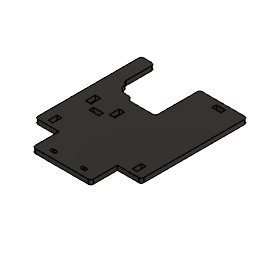
つくプロ (Autodesk Fusion 360 design; units mm, degrees)
Autodesk Fusion 360 part; units mm, degrees
sketch "スケッチ1" plane through (0, 0, 0) normal (0, 0, 1) x (1, 0, 0)
  line L0 (-60, 15) -> (-60, 150)
  line L1 (0, 165) -> (0, 0)
  line L2 (60, 15) -> (60, 150)
  line L3 (-60, 150) -> (-60, 165)
  line L4 (-60, 165) -> (60, 165)
  line L5 (60, 165) -> (60, 150)
  line L6 (-60, 15) -> (60, 15)
  dimension "d20" = 15
  constraint vertical L0
  constraint vertical L1
  constraint coincident L1.end origin
  constraint symmetric L0.end L1 L2.end
  constraint vertical L3
  constraint horizontal L4
  constraint vertical L5
  constraint midpoint L1.start L4
  constraint horizontal L6
  measures "d20" distance of L2.end L4.end
extrude "押し出し1" add sketch "スケッチ1" along normal blind 5
sketch "スケッチ2" plane through (0, 0, 5) normal (0, 0, 1) x (-1, 0, 0)
  line L0 (-60, -15) -> (-60, -165)
  line L1 (60, -165) -> (60, -15)
  line L2 (60, -15) -> (33, -15)
  line L3 (33, -15) -> (33, -45)
  line L4 (33, -45) -> (60, -45)
  line L5 (60, -45) -> (60, -15)
  line L6 (0, -150) -> (0, 0)
  line L7 (-33, -45) -> (-60, -45)
  line L8 (-60, -45) -> (-60, -15)
  line L9 (-60, -15) -> (-33, -15)
  line L10 (-33, -15) -> (-33, -45)
  line L11 (45, -73.5175) -> (45, 1.4825)
  line L12 (60, -15) -> (-60, -15)
  line L13 (-60, -165) -> (60, -165)
  dimension "d38" = 27
  constraint horizontal L2
  constraint vertical L3
  constraint horizontal L4
  constraint vertical L5
  constraint coincident L1 L2.start
  constraint coincident L6.end origin
  constraint symmetric L1.end L6 L0.start
  constraint symmetric L2.end L6 L9.end
  measures "d38" distance of L3 L5
extrude "押し出し2" cut sketch "スケッチ2" against normal blind 35 contours L0 L7 L8 L9 L10 L12 | L2 L3 L4 L11 L12 | L1 L2 L4 L5 L11 L12
fillet "フィレット1" radius 3 6 edges at (60, 45, 2.5) (60, 165, 2.5) (-60, 165, 2.5) (-60, 45, 2.5) (-33, 15, 2.5) (33, 15, 2.5)
sketch "スケッチ16" plane through (0, 0, 5) normal (0, 0, 1) x (-1, 0, 0)
  arc A0 (-30, -15) -> (-33, -18) centre (-30, -18) ccw
  line L0 (-33, -18) -> (-33, -45)
  line L1 (-33, -45) -> (-57, -45)
  arc A1 (-57, -45) -> (-60, -48) centre (-57, -48) ccw
  line L2 (-60, -48) -> (-60, -162)
  arc A2 (-60, -162) -> (-57, -165) centre (-57, -162) ccw
  line L3 (-57, -165) -> (57, -165)
  arc A3 (57, -165) -> (60, -162) centre (57, -162) ccw
  line L4 (60, -162) -> (60, -48)
  arc A4 (60, -48) -> (57, -45) centre (57, -48) ccw
  line L5 (57, -45) -> (33, -45)
  line L6 (33, -45) -> (33, -18)
  arc A5 (33, -18) -> (30, -15) centre (30, -18) ccw
  line L7 (30, -15) -> (-30, -15)
  line L8 (45, -140) -> (25, -140)
  line L9 (25, -140) -> (25, -100)
  line L10 (25, -100) -> (45, -100)
  line L11 (45, -100) -> (45, -140)
  circle A6 centre (31.5, -129.6605) radius 10.3395
  circle A7 centre (31.5, -129.6605) radius 37.5
  line L12 (-6, -100) -> (-6, -146)
  line L13 (-6, -100) -> (25, -100)
  line L14 (25, -115) -> (-6, -115)
  line L15 (25, -165) -> (45, -165)
  line L16 (45, -165) -> (45, -140)
  line L17 (45, -140) -> (25, -140)
  line L18 (25, -140) -> (25, -165)
  line L19 (31.5, -129.6605) -> (45, -129.6605)
  line L20 (25, -165) -> (-6, -165)
  line L21 (-6, -165) -> (-6, -146)
  line L22 (-6, -146) -> (25, -146)
  line L23 (25, -146) -> (25, -165)
  dimension "d49" = 40
  dimension "d50" = 20
  dimension "d51" = 25
  dimension "d52" = 15
  dimension "d53" = 75
  dimension "d54" = 65
  constraint horizontal L8
  constraint vertical L9
  constraint horizontal L10
  constraint vertical L11
  constraint tangent L8 A6
  constraint concentric A6 A7
  constraint vertical L12
  constraint tangent A7 L12
  constraint coincident L9 L14.start
  constraint coincident L12 L14.end
  constraint perpendicular L12 L14
  constraint horizontal L15
  constraint vertical L16
  constraint horizontal L17
  constraint vertical L18
  constraint coincident L3 L15.start
  constraint coincident A6.centre A7.centre
  constraint coincident L11 L19.end
  constraint perpendicular L11 L19
  constraint horizontal L20
  constraint vertical L21
  constraint horizontal L22
  constraint vertical L23
  measures "d49" distance of L8.start L10.end
  measures "d50" distance of L9.end L10.end
  measures "d51" distance of L3 L8
  measures "d52" distance of L4 L11
  measures "d53" diameter of A7
  measures "d54" distance of L3 L12.start
extrude "押し出し12" cut sketch "スケッチ16" against normal blind 5 contours L3 A7 L20 L21 L22 | L3 A7 L18 L20 L22 L23 | A7 L12 L22 | L3 A7 L15 L16 | L3 L8 A7 L15 L16 L17 L18 L23 | L9 A6 A7 L14 L18 L22 | A7 L12 L14 | L8 L11 A6 L17 L19 | L8 L9 A6 L17 | L9 A6 | L9 A6
sketch "スケッチ17" plane through (0, 0, 5) normal (0, 0, 1) x (-1, 0, 0)
  line L0 (-6, -165) -> (-6, -115)
  line L1 (-6, -115) -> (25, -115)
  line L2 (25, -115) -> (25, -121.6196)
  arc A0 (41.8395, -129.6605) -> (25, -121.6196) centre (31.5, -129.6605) ccw
  line L3 (41.8395, -129.6605) -> (45, -129.6605)
  line L4 (45, -129.6605) -> (45, -165)
  line L5 (45, -165) -> (57, -165)
  arc A1 (57, -165) -> (60, -162) centre (57, -162) ccw
  line L6 (60, -162) -> (60, -48)
  arc A2 (60, -48) -> (57, -45) centre (57, -48) ccw
  line L7 (57, -45) -> (33, -45)
  line L8 (33, -45) -> (33, -18)
  arc A3 (33, -18) -> (30, -15) centre (30, -18) ccw
  line L9 (30, -15) -> (-30, -15)
  arc A4 (-30, -15) -> (-33, -18) centre (-30, -18) ccw
  line L10 (-33, -18) -> (-33, -45)
  line L11 (-33, -45) -> (-57, -45)
  arc A5 (-57, -45) -> (-60, -48) centre (-57, -48) ccw
  line L12 (-60, -48) -> (-60, -162)
  line L13 (-57, -165) -> (-6, -165)
  line L14 (-40, -23) -> (40, -23)
  circle A6 centre (-17, -23) radius 1.65
  line L15 (-18.65, -24.65) -> (-15.35, -24.65)
  line L16 (-15.35, -24.65) -> (-15.35, -21.35)
  line L17 (-15.35, -21.35) -> (-18.65, -21.35)
  line L18 (-18.65, -21.35) -> (-18.65, -24.65)
  line L19 (0, 0) -> (0, -40)
  circle A7 centre (-18.65, -23) radius 1.65
  circle A8 centre (-15.35, -23) radius 1.65
  line L20 (18.65, -21.35) -> (18.65, -24.65)
  line L21 (15.35, -21.35) -> (18.65, -21.35)
  line L22 (18.65, -24.65) -> (15.35, -24.65)
  circle A9 centre (15.35, -23) radius 1.65
  line L23 (15.35, -24.65) -> (15.35, -21.35)
  circle A10 centre (18.65, -23) radius 1.65
  point P0 (17, -23)
  dimension "d57" = 8
  dimension "d58" = 16
  dimension "d61" = 3.3
  constraint perpendicular L8 L14
  constraint coincident L14 A6.centre
  constraint horizontal L15
  constraint vertical L16
  constraint horizontal L17
  constraint vertical L18
  constraint tangent A6 L15
  constraint tangent A6 L17
  constraint tangent A6 L18
  constraint tangent A6 L16
  constraint coincident L19.start origin
  constraint vertical L19
  constraint midpoint L18 A7.centre
  constraint coincident L15.start A7
  constraint midpoint L16 A8.centre
  constraint coincident L15.end A8
  constraint symmetric A6.centre L19 P0
  constraint symmetric L15.start L19 L20.end
  constraint symmetric L15.end L19 L22.end
  constraint symmetric L16.end L19 L21.start
  constraint symmetric L17.end L19 L20.start
  constraint symmetric L19 A7 A10
  constraint symmetric L19 A8 A9
  measures "d57" distance of L9 L14
  measures "d58" distance of L10 A6.centre
  measures "d61" diameter of A6
extrude "押し出し13" cut sketch "スケッチ17" against normal blind 6 contours L14 L20 A10 | L14 L20 A10 | L14 L20 A10 | L14 L20 A10 | L21 A9 A10 | L22 A9 A10 | L14 A9 L23 | L14 A9 L23 | L14 A9 L23 | L14 A9 L23 | L14 L16 A8 | L14 L16 A8 | L14 A6 A8 | L14 A6 A8 | A6 L16 A8 | A6 L16 A8 | A6 L17 A8 | A6 L15 A8 | L14 L18 A7 | L14 L18 A7 | L14 A6 A7 | L14 A6 A7 | A6 A7 A8 | A6 A7 A8 | A6 L17 A7 | A6 L15 A7 | A6 L18 A7 | A6 L18 A7
sketch "スケッチ18" plane through (0, 0, 5) normal (0, 0, 1) x (-1, 0, 0)
  line L0 (18.65, -24.65) -> (15.35, -24.65)
  arc A0 (15.35, -21.35) -> (15.35, -24.65) centre (15.35, -23) ccw
  line L1 (15.35, -21.35) -> (18.65, -21.35)
  arc A1 (18.65, -24.65) -> (18.65, -21.35) centre (18.65, -23) ccw
  line L2 (-18.65, -21.35) -> (-15.35, -21.35)
  arc A2 (-15.35, -24.65) -> (-15.35, -21.35) centre (-15.35, -23) ccw
  line L3 (-15.35, -24.65) -> (-18.65, -24.65)
  arc A3 (-18.65, -21.35) -> (-18.65, -24.65) centre (-18.65, -23) ccw
  line L4 (-6, -165) -> (-6, -115)
  line L5 (-6, -115) -> (25, -115)
  line L6 (25, -115) -> (25, -121.6196)
  arc A4 (41.8395, -129.6605) -> (25, -121.6196) centre (31.5, -129.6605) ccw
  line L7 (41.8395, -129.6605) -> (45, -129.6605)
  line L8 (45, -129.6605) -> (45, -165)
  line L9 (45, -165) -> (57, -165)
  arc A5 (57, -165) -> (60, -162) centre (57, -162) ccw
  line L10 (60, -162) -> (60, -48)
  arc A6 (60, -48) -> (57, -45) centre (57, -48) ccw
  line L11 (57, -45) -> (33, -45)
  line L12 (33, -45) -> (33, -18)
  arc A7 (33, -18) -> (30, -15) centre (30, -18) ccw
  line L13 (30, -15) -> (-30, -15)
  arc A8 (-30, -15) -> (-33, -18) centre (-30, -18) ccw
  line L14 (-33, -18) -> (-33, -45)
  line L15 (-33, -45) -> (-57, -45)
  arc A9 (-57, -45) -> (-60, -48) centre (-57, -48) ccw
  line L16 (-60, -48) -> (-60, -162)
  arc A10 (-60, -162) -> (-57, -165) centre (-57, -162) ccw
  line L17 (-57, -165) -> (-6, -165)
  line L18 (25, -119.3209) -> (37, -119.3209)
  constraint coincident L6 L18.start
  constraint perpendicular L6 L18
  constraint tangent A4 L18
extrude "押し出し14" cut sketch "スケッチ18" against normal blind 11 contours L6 A4 L18
sketch "スケッチ19" plane through (0, 0, 0) normal (0, 0, -1) x (1, 0, 0)
  line L0 (-31.5, -119.3209) -> (-25, -119.3209)
  line L1 (-25, -119.3209) -> (-25, -115)
  line L2 (-25, -115) -> (6, -115)
  line L3 (6, -115) -> (6, -165)
  line L4 (6, -165) -> (57, -165)
  arc A0 (57, -165) -> (60, -162) centre (57, -162) ccw
  line L5 (60, -162) -> (60, -48)
  arc A1 (60, -48) -> (57, -45) centre (57, -48) ccw
  line L6 (57, -45) -> (33, -45)
  line L7 (33, -45) -> (33, -18)
  arc A2 (33, -18) -> (30, -15) centre (30, -18) ccw
  line L8 (30, -15) -> (-30, -15)
  arc A3 (-30, -15) -> (-33, -18) centre (-30, -18) ccw
  line L9 (-33, -18) -> (-33, -45)
  line L10 (-33, -45) -> (-57, -45)
  arc A4 (-57, -45) -> (-60, -48) centre (-57, -48) ccw
  line L11 (-60, -48) -> (-60, -162)
  arc A5 (-60, -162) -> (-57, -165) centre (-57, -162) ccw
  line L12 (-57, -165) -> (-45, -165)
  line L13 (-45, -165) -> (-45, -129.6605)
  line L14 (-45, -129.6605) -> (-41.8395, -129.6605)
  arc A6 (-31.5, -119.3209) -> (-41.8395, -129.6605) centre (-31.5, -129.6605) ccw
  line L15 (15.35, -21.35) -> (18.65, -21.35)
  arc A7 (18.65, -24.65) -> (18.65, -21.35) centre (18.65, -23) ccw
  line L16 (18.65, -24.65) -> (15.35, -24.65)
  arc A8 (15.35, -21.35) -> (15.35, -24.65) centre (15.35, -23) ccw
  line L17 (-15.35, -24.65) -> (-18.65, -24.65)
  arc A9 (-18.65, -21.35) -> (-18.65, -24.65) centre (-18.65, -23) ccw
  line L18 (-18.65, -21.35) -> (-15.35, -21.35)
  arc A10 (-15.35, -24.65) -> (-15.35, -21.35) centre (-15.35, -23) ccw
  line L19 (-65, -100.66) -> (65, -100.66)
  line L20 (-47.5, -90) -> (-47.5, -113.3169)
  line L21 (-47.5, -100.66) -> (-42.5, -100.66)
  line L22 (-42.5, -100.66) -> (-42.5, -90.66)
  line L23 (-42.5, -90.66) -> (-47.5, -90.66)
  line L24 (-47.5, -90.66) -> (-47.5, -100.66)
  line L25 (-48, -101.16) -> (-42, -101.16)
  line L26 (-42, -101.16) -> (-42, -90.16)
  line L27 (-42, -90.16) -> (-48, -90.16)
  line L28 (-48, -90.16) -> (-48, -101.16)
  line L29 (-36.5, -87.66) -> (-31.5, -87.66)
  line L30 (-31.5, -87.66) -> (-31.5, -83.66)
  line L31 (-31.5, -83.66) -> (-36.5, -83.66)
  line L32 (-36.5, -83.66) -> (-36.5, -87.66)
  line L33 (-31.5, -88.16) -> (-37, -88.16)
  line L34 (-37, -88.16) -> (-37, -83.16)
  line L35 (-37, -83.16) -> (-31.5, -83.16)
  line L36 (-31.5, -83.16) -> (-31.5, -88.16)
  line L37 (-15, -90.16) -> (-15, -101.16)
  line L38 (-21, -90.16) -> (-15, -90.16)
  line L39 (-21, -101.16) -> (-21, -90.16)
  line L40 (-15, -101.16) -> (-21, -101.16)
  line L41 (-26, -83.16) -> (-31.5, -83.16)
  line L42 (-26, -88.16) -> (-26, -83.16)
  line L43 (-31.5, -88.16) -> (-26, -88.16)
  dimension "d68" = 64.34
  dimension "d69" = 12.5
  dimension "d70" = 5
  dimension "d71" = 10
  dimension "d72" = 6
  dimension "d73" = 11
  dimension "d74" = 0.5
  dimension "d75" = 0.5
  dimension "d78" = 4
  dimension "d79" = 5
  dimension "d80" = 11
  dimension "d81" = 5
  dimension "d82" = 5.5
  dimension "d83" = 3
  dimension "d84" = 0.5
  dimension "d85" = 0.5
  constraint perpendicular L5 L19
  constraint parallel L11 L20
  constraint horizontal L21
  constraint vertical L22
  constraint horizontal L23
  constraint vertical L24
  constraint coincident L20 L21.start
  constraint coincident L19 L21.start
  constraint horizontal L25
  constraint vertical L26
  constraint horizontal L27
  constraint vertical L28
  constraint horizontal L29
  constraint vertical L30
  constraint horizontal L31
  constraint vertical L32
  constraint horizontal L33
  constraint vertical L34
  constraint horizontal L35
  constraint vertical L36
  constraint symmetric L25.start L36 L37.end
  constraint symmetric L25.end L36 L39.start
  constraint symmetric L26.end L36 L38.start
  constraint symmetric L27.end L36 L37.start
  constraint symmetric L33.start L36 L43.start
  constraint symmetric L33.end L36 L42.start
  constraint symmetric L34.end L36 L41.start
  constraint symmetric L35.end L36 L41.end
  measures "d68" distance of L12 L19
  measures "d69" distance of L11 L20
  measures "d70" distance of L22.end L23.end
  measures "d71" distance of L21.start L23.end
  measures "d72" distance of L26.end L27.end
  measures "d73" distance of L25.end L26.end
  measures "d74" distance of L23 L27
  measures "d75" distance of L22 L26
  measures "d78" distance of L29.start L31.end
  measures "d79" distance of L30.end L31.end
  measures "d80" distance of L24 L32
  measures "d81" distance of L33.end L34.end
  measures "d82" distance of L34.end L35.end
  measures "d83" distance of L23 L29
  measures "d84" distance of L31 L35
  measures "d85" distance of L32 L34
extrude "押し出し15" cut sketch "スケッチ19" against normal blind 16 contours L19 L20 L24 L27 L28 | L19 L20 L25 L28 | L19 L37 L39 L40 | L19 L37 L38 L39 | L19 L20 L21 L22 L23 L24 | L19 L20 L21 L25 L26 | L19 L20 L22 L23 L26 L27 | L29 L30 L31 L32 L36 | L29 L31 L32 L33 L34 L35 L36 | L30 L36 L41 L42 L43
fillet "フィレット2" radius 3 4 edges at (6, 115, 2.5) (-25, 119.3209, 2.5) (6, 165, 2.5) (-45, 165, 2.5)
fillet "フィレット2" radius 3 3 edges at (-41.8395, 129.6605, 2.5) (-45, 129.6605, 2.5) (-25, 115, 2.5)
sketch "スケッチ20" plane through (0, 0, 0) normal (0, 0, -1) x (1, 0, 0)
  arc A0 (-43.3112, -129.9622) -> (-41.6713, -127.8029) centre (-44.6225, -127.2639) ccw
  arc A1 (-31.5, -119.3209) -> (-41.6713, -127.8029) centre (-31.5, -129.6605) ccw
  line L0 (-31.5, -119.3209) -> (-28, -119.3209)
  arc A2 (-28, -119.3209) -> (-25.1199, -117.1605) centre (-28, -116.3209) ccw
  arc A3 (-22.2397, -115) -> (-25.1199, -117.1605) centre (-22.2397, -118) ccw
  line L1 (-22.2397, -115) -> (3, -115)
  arc A4 (6, -118) -> (3, -115) centre (3, -118) ccw
  line L2 (6, -118) -> (6, -162)
  arc A5 (6, -162) -> (9, -165) centre (9, -162) ccw
  line L3 (9, -165) -> (57, -165)
  arc A6 (57, -165) -> (60, -162) centre (57, -162) ccw
  line L4 (60, -162) -> (60, -48)
  arc A7 (60, -48) -> (57, -45) centre (57, -48) ccw
  line L5 (57, -45) -> (33, -45)
  line L6 (33, -45) -> (33, -18)
  arc A8 (33, -18) -> (30, -15) centre (30, -18) ccw
  line L7 (30, -15) -> (-30, -15)
  arc A9 (-30, -15) -> (-33, -18) centre (-30, -18) ccw
  line L8 (-33, -18) -> (-33, -45)
  line L9 (-33, -45) -> (-57, -45)
  arc A10 (-57, -45) -> (-60, -48) centre (-57, -48) ccw
  line L10 (-60, -48) -> (-60, -162)
  arc A11 (-60, -162) -> (-57, -165) centre (-57, -162) ccw
  line L11 (-57, -165) -> (-48, -165)
  arc A12 (-48, -165) -> (-45, -162) centre (-48, -162) ccw
  line L12 (-45, -162) -> (-45, -132.6605)
  arc A13 (-43.3112, -129.9622) -> (-45, -132.6605) centre (-42, -132.6605) ccw
  line L13 (-15.35, -24.65) -> (-18.65, -24.65)
  arc A14 (-18.65, -21.35) -> (-18.65, -24.65) centre (-18.65, -23) ccw
  line L14 (-18.65, -21.35) -> (-15.35, -21.35)
  arc A15 (-15.35, -24.65) -> (-15.35, -21.35) centre (-15.35, -23) ccw
  line L15 (15.35, -21.35) -> (18.65, -21.35)
  arc A16 (18.65, -24.65) -> (18.65, -21.35) centre (18.65, -23) ccw
  line L16 (18.65, -24.65) -> (15.35, -24.65)
  arc A17 (15.35, -21.35) -> (15.35, -24.65) centre (15.35, -23) ccw
  line L17 (-21, -90.16) -> (-15, -90.16)
  line L18 (-15, -90.16) -> (-15, -101.16)
  line L19 (-15, -101.16) -> (-21, -101.16)
  line L20 (-21, -101.16) -> (-21, -90.16)
  line L21 (-26, -83.16) -> (-26, -88.16)
  line L22 (-26, -88.16) -> (-37, -88.16)
  line L23 (-37, -88.16) -> (-37, -83.16)
  line L24 (-37, -83.16) -> (-26, -83.16)
  line L25 (-42, -101.16) -> (-48, -101.16)
  line L26 (-48, -101.16) -> (-48, -90.16)
  line L27 (-48, -90.16) -> (-42, -90.16)
  line L28 (-42, -90.16) -> (-42, -101.16)
  line L29 (-50, -60) -> (-45, -60)
  line L30 (-45, -60) -> (-45, -50)
  line L31 (-45, -50) -> (-50, -50)
  line L32 (-50, -50) -> (-50, -60)
  line L33 (30, -160) -> (40, -160)
  line L34 (40, -160) -> (40, -155)
  line L35 (40, -155) -> (30, -155)
  line L36 (30, -155) -> (30, -160)
  line L37 (0, -10) -> (0, 10)
  line L38 (45, -50) -> (50, -50)
  line L39 (45, -60) -> (45, -50)
  line L40 (50, -50) -> (50, -60)
  line L41 (50, -60) -> (45, -60)
  constraint horizontal L29
  constraint vertical L30
  constraint horizontal L31
  constraint vertical L32
  constraint horizontal L33
  constraint vertical L34
  constraint horizontal L35
  constraint vertical L36
  constraint perpendicular L7 L37
  constraint symmetric L29.start L37 L40.end
  constraint symmetric L29.end L37 L39.start
  constraint symmetric L30.end L37 L38.start
  constraint symmetric L31.end L37 L38.end
extrude "押し出し16" cut sketch "スケッチ20" against normal blind 20 contours L29 L30 L31 L32 | L33 L34 L35 L36 | L38 L39 L40 L41
